Autodesk Fusion 360 part; units mm, degrees
(part 2 of 11)
  line L821 (19.8574, -105.4367) -> (19.8738, -105.4005)
  line L822 (-0.0787, -205.2079) -> (-0.0748, -205.2474)
  arc A58 (18.12, -106.7368) -> (18.4614, -106.8782) centre (18.32, -106.7368) ccw
  line L823 (0.0706, -205.5685) -> (0.0978, -205.5975)
  line L824 (19.7422, -105.5975) -> (19.7694, -105.5685)
  line L825 (0.0454, -45.5378) -> (0.0706, -45.5685)
  line L826 (19.9083, -105.2866) -> (19.9148, -105.2474)
  line L827 (-0.0338, -205.4005) -> (-0.0174, -205.4367)
  line L828 (19.7694, -105.5685) -> (19.7946, -105.5378)
  line L829 (1.72, -46.7368) -> (1.72, -44.4997)
  line L830 (19.9187, -105.2079) -> (19.92, -105.0997)
  line L831 (-0.0683, -45.2866) -> (-0.0593, -45.3253)
  arc A59 (1.3786, -46.8782) -> (1.72, -46.7368) centre (1.52, -46.7368) ccw
  line L832 (0.0706, -45.5685) -> (0.0978, -45.5975)
  line L833 (19.8387, -105.4717) -> (19.8574, -105.4367)
  line L834 (0.0454, -205.5378) -> (0.0706, -205.5685)
  line L835 (19.9148, -105.2474) -> (19.9187, -105.2079)
  line L836 (-0.0683, -205.2866) -> (-0.0593, -205.3253)
  line L837 (0.0223, -45.5055) -> (0.0454, -45.5378)
  line L838 (-0.0683, -45.2866) -> (-0.0593, -45.3253)
  line L839 (-0.0593, -45.3253) -> (-0.0478, -45.3633)
  line L840 (-0.0478, -185.3633) -> (-0.0338, -185.4005)
  line L841 (6.02, -189.7998) -> (6.2199, -189.9997)
  line L842 (9.713, -186.0997) -> (7.0807, -186.0997)
  line L843 (-0.0787, -205.2079) -> (-0.0748, -205.2474)
  line L844 (-0.0174, -45.4367) -> (0.0013, -45.4717)
  line L845 (19.9187, -105.2079) -> (19.92, -105.0997)
  line L846 (0.0706, -205.5685) -> (0.0978, -205.5975)
  line L847 (-0.0593, -45.3253) -> (-0.0478, -45.3633)
  line L848 (0.0454, -205.5378) -> (0.0706, -205.5685)
  line L849 (19.8993, -105.3253) -> (19.9083, -105.2866)
  line L850 (0.0223, -205.5055) -> (0.0454, -205.5378)
  line L851 (-0.0338, -205.4005) -> (-0.0174, -205.4367)
  line L852 (19.8177, -105.5055) -> (19.8387, -105.4717)
  line L853 (6.02, -187.1603) -> (6.02, -189.7998)
  line L854 (0.0013, -45.4717) -> (0.0223, -45.5055)
  line L855 (0.0223, -185.5055) -> (0.0454, -185.5378)
  line L856 (9.92, -186.3066) -> (9.713, -186.0997)
  line L857 (-0.0478, -45.3633) -> (-0.0338, -45.4005)
  line L858 (-0.08, -45.0997) -> (-0.0787, -45.2079)
  line L859 (19.8387, -105.4717) -> (19.8574, -105.4367)
  line L860 (0.0013, -205.4717) -> (0.0223, -205.5055)
  line L861 (19.7946, -105.5378) -> (19.8177, -105.5055)
  line L862 (19.9148, -105.2474) -> (19.9187, -105.2079)
  line L863 (19.8738, -105.4005) -> (19.8878, -105.3633)
  line L864 (1.72, -206.7368) -> (1.72, -204.4997)
  line L865 (-0.0593, -205.3253) -> (-0.0478, -205.3633)
  line L866 (19.8878, -105.3633) -> (19.8993, -105.3253)
  line L867 (19.8177, -105.5055) -> (19.8387, -105.4717)
  line L868 (-0.08, -185.0997) -> (-0.0787, -185.2079)
  line L869 (0.0013, -45.4717) -> (0.0223, -45.5055)
  line L870 (19.9083, -105.2866) -> (19.9148, -105.2474)
  line L871 (-0.0683, -205.2866) -> (-0.0593, -205.3253)
  line L872 (-0.0748, -205.2474) -> (-0.0683, -205.2866)
  line L873 (-0.0787, -45.2079) -> (-0.0748, -45.2474)
  line L874 (-0.0174, -205.4367) -> (0.0013, -205.4717)
  line L875 (18.4614, -106.8782) -> (19.7422, -105.5975)
  line L876 (-0.0174, -45.4367) -> (0.0013, -45.4717)
  line L877 (-0.0748, -205.2474) -> (-0.0683, -205.2866)
  line L878 (18.12, -97.2997) -> (18.12, -102.6997)
  line L879 (-0.08, -205.0997) -> (-0.0787, -205.2079)
  arc A60 (1.3786, -46.8782) -> (1.72, -46.7368) centre (1.52, -46.7368) ccw
  line L880 (10.127, -206.0997) -> (9.92, -206.3066)
  line L881 (-0.0593, -94.674) -> (-0.0683, -94.7127)
  line L882 (9.713, -193.8997) -> (9.92, -193.6927)
  circle A61 centre (9.92, -49.9997) radius 2.1
  line L883 (19.8878, -105.3633) -> (19.8993, -105.3253)
  line L884 (0.0223, -94.4938) -> (0.0013, -94.5276)
  line L885 (9.713, -206.0997) -> (7.0807, -206.0997)
  line L886 (10.127, -193.8997) -> (12.7593, -193.8997)
  line L887 (3.6807, -197.2997) -> (7.0807, -193.8997)
  line L888 (9.92, -193.6927) -> (10.127, -193.8997)
  line L889 (9.92, -206.3066) -> (9.713, -206.0997)
  line L890 (18.12, -102.6997) -> (16.1593, -102.6997)
  line L891 (16.4807, -104.4997) -> (18.12, -104.4997)
  line L892 (-0.0338, -45.4005) -> (-0.0174, -45.4367)
  line L893 (13.82, -107.1603) -> (16.4807, -104.4997)
  line L894 (7.0807, -206.0997) -> (3.6807, -202.6997)
  line L895 (7.0807, -193.8997) -> (9.713, -193.8997)
  line L896 (9.92, -206.3066) -> (9.713, -206.0997)
  line L897 (7.0807, -193.8997) -> (9.713, -193.8997)
  line L898 (19.8993, -105.3253) -> (19.9083, -105.2866)
  line L899 (-0.0174, -205.4367) -> (0.0013, -205.4717)
  line L900 (-0.08, -45.0997) -> (-0.0787, -45.2079)
  line L901 (0.0978, -45.5975) -> (1.3786, -46.8782)
  line L902 (6.02, -192.839) -> (3.3593, -195.4997)
  line L903 (10.127, -193.8997) -> (12.7593, -193.8997)
  line L904 (12.7593, -106.0997) -> (10.127, -106.0997)
  line L905 (-0.0338, -45.4005) -> (-0.0174, -45.4367)
  line L906 (0.0978, -45.5975) -> (1.3786, -46.8782)
  line L907 (-0.0748, -45.2474) -> (-0.0683, -45.2866)
  line L908 (13.82, -107.1603) -> (16.4807, -104.4997)
  line L909 (0.0013, -205.4717) -> (0.0223, -205.5055)
  line L910 (18.12, -97.2997) -> (18.12, -102.6997)
  line L911 (13.82, -109.7998) -> (13.82, -107.1603)
  line L912 (16.1593, -97.2997) -> (18.12, -97.2997)
  line L913 (-0.0478, -205.3633) -> (-0.0338, -205.4005)
  line L914 (0.0223, -45.5055) -> (0.0454, -45.5378)
  line L915 (18.12, -104.4997) -> (18.12, -106.7368)
  line L916 (16.1593, -102.6997) -> (12.7593, -106.0997)
  line L917 (-0.0478, -205.3633) -> (-0.0338, -205.4005)
  line L918 (-0.0478, -45.3633) -> (-0.0338, -45.4005)
  line L919 (18.12, -104.4997) -> (18.12, -106.7368)
  line L920 (6.02, -192.839) -> (3.3593, -195.4997)
  line L921 (19.7422, -105.5975) -> (19.7694, -105.5685)
  line L922 (12.7593, -106.0997) -> (10.127, -106.0997)
  line L923 (9.92, -193.6927) -> (10.127, -193.8997)
  line L924 (9.713, -193.8997) -> (9.92, -193.6927)
  line L925 (9.713, -206.0997) -> (7.0807, -206.0997)
  line L926 (12.7593, -206.0997) -> (10.127, -206.0997)
  line L927 (10.127, -206.0997) -> (9.92, -206.3066)
  line L928 (12.7593, -206.0997) -> (10.127, -206.0997)
  line L929 (13.82, -109.7998) -> (13.82, -107.1603)
  line L930 (-0.08, -194.8997) -> (-0.08, -205.0997)
  line L931 (-0.08, -194.8997) -> (-0.08, -205.0997)
  line L932 (18.12, -102.6997) -> (16.1593, -102.6997)
  line L933 (-0.0748, -45.2474) -> (-0.0683, -45.2866)
  line L934 (16.4807, -104.4997) -> (18.12, -104.4997)
  line L935 (16.1593, -97.2997) -> (18.12, -97.2997)
  line L936 (16.1593, -102.6997) -> (12.7593, -106.0997)
  line L937 (6.02, -47.1603) -> (6.02, -49.7998)
  line L938 (3.6807, -197.2997) -> (7.0807, -193.8997)
  line L939 (-0.0748, -94.7519) -> (-0.0787, -94.7914)
  line L940 (-0.0338, -94.5988) -> (-0.0478, -94.636)
  line L941 (3.3593, -95.4997) -> (1.72, -95.4997)
  line L942 (3.3593, -95.4997) -> (1.72, -95.4997)
  line L943 (-0.0593, -94.674) -> (-0.0683, -94.7127)
  line L944 (1.72, -204.4997) -> (3.3593, -204.4997)
  line L945 (1.72, -204.4997) -> (3.3593, -204.4997)
  line L946 (0.0706, -94.4308) -> (0.0454, -94.4616)
  line L947 (1.72, -197.2997) -> (3.6807, -197.2997)
  line L948 (3.6807, -202.6997) -> (1.72, -202.6997)
  line L949 (3.6807, -202.6997) -> (1.72, -202.6997)
  line L950 (0.0223, -94.4938) -> (0.0013, -94.5276)
  line L951 (0.0013, -94.5276) -> (-0.0174, -94.5626)
  line L952 (7.0807, -206.0997) -> (3.6807, -202.6997)
  line L953 (0.0223, -85.5055) -> (0.0454, -85.5378)
  line L954 (9.713, -53.8997) -> (9.92, -53.6927)
  line L955 (19.8738, -194.5988) -> (19.8574, -194.5626)
  arc A62 (1.3786, -86.8782) -> (1.72, -86.7368) centre (1.52, -86.7368) ccw
  line L956 (7.0807, -86.0997) -> (4.42, -83.439)
  line L957 (9.92, -53.6927) -> (10.127, -53.8997)
  line L958 (19.8574, -194.5626) -> (19.8387, -194.5276)
  line L959 (18.12, -204.4997) -> (18.12, -206.7368)
  line L960 (1.72, -84.4997) -> (3.3593, -84.4997)
  line L961 (0.0223, -85.5055) -> (0.0454, -85.5378)
  line L962 (7.0807, -86.0997) -> (4.42, -83.439)
  line L963 (19.8738, -194.5988) -> (19.8574, -194.5626)
  line L964 (-0.0748, -85.2474) -> (-0.0683, -85.2866)
  line L965 (-0.0338, -85.4005) -> (-0.0174, -85.4367)
  line L966 (19.7694, -194.4308) -> (19.7422, -194.4019)
  line L967 (19.9187, -194.7914) -> (19.9148, -194.7519)
  line L968 (0.0706, -85.5685) -> (0.0978, -85.5975)
  line L969 (-0.0338, -85.4005) -> (-0.0174, -85.4367)
  line L970 (3.3593, -84.4997) -> (6.02, -87.1603)
  line L971 (16.4807, -204.4997) -> (18.12, -204.4997)
  line L972 (9.92, -53.6927) -> (10.127, -53.8997)
  line L973 (19.9187, -205.2079) -> (19.92, -205.0997)
  line L974 (19.8738, -205.4005) -> (19.8878, -205.3633)
  line L975 (6.02, -52.839) -> (3.3593, -55.4997)
  line L976 (-0.0683, -85.2866) -> (-0.0593, -85.3253)
  line L977 (3.3593, -44.4997) -> (6.02, -47.1603)
  line L978 (-0.0478, -85.3633) -> (-0.0338, -85.4005)
  line L979 (19.9148, -194.7519) -> (19.9083, -194.7127)
  line L980 (18.12, -197.2997) -> (18.12, -202.6997)
  line L981 (0.0454, -85.5378) -> (0.0706, -85.5685)
  line L982 (18.12, -202.6997) -> (16.1593, -202.6997)
  line L983 (19.7946, -194.4616) -> (19.7694, -194.4308)
  line L984 (18.12, -202.6997) -> (16.1593, -202.6997)
  line L985 (6.02, -52.839) -> (3.3593, -55.4997)
  line L986 (6.02, -49.7998) -> (6.2199, -49.9997)
  line L987 (-0.0787, -85.2079) -> (-0.0748, -85.2474)
  arc A63 (1.3786, -86.8782) -> (1.72, -86.7368) centre (1.52, -86.7368) ccw
  line L988 (-0.0748, -85.2474) -> (-0.0683, -85.2866)
  line L989 (3.6807, -57.2997) -> (7.0807, -53.8997)
  line L990 (6.2199, -49.9997) -> (6.02, -50.1995)
  line L991 (-0.08, -85.0997) -> (-0.0787, -85.2079)
  line L992 (0.0706, -85.5685) -> (0.0978, -85.5975)
  line L993 (-0.0593, -85.3253) -> (-0.0478, -85.3633)
  line L994 (18.12, -197.2997) -> (18.12, -202.6997)
  line L995 (7.0807, -53.8997) -> (9.713, -53.8997)
  line L996 (10.127, -46.0997) -> (9.92, -46.3066)
  line L997 (0.0013, -85.4717) -> (0.0223, -85.5055)
  line L998 (16.1593, -197.2997) -> (18.12, -197.2997)
  line L999 (7.0807, -53.8997) -> (9.713, -53.8997)
  line L1000 (1.72, -84.4997) -> (3.3593, -84.4997)
  line L1001 (3.3593, -44.4997) -> (6.02, -47.1603)
  line L1002 (-0.0174, -85.4367) -> (0.0013, -85.4717)
  line L1003 (0.0454, -85.5378) -> (0.0706, -85.5685)
  line L1004 (18.12, -193.2625) -> (18.12, -195.4997)
  line L1005 (19.9083, -194.7127) -> (19.8993, -194.674)
  line L1006 (-0.0787, -85.2079) -> (-0.0748, -85.2474)
  line L1007 (-0.0174, -85.4367) -> (0.0013, -85.4717)
  line L1008 (16.1593, -197.2997) -> (18.12, -197.2997)
  line L1009 (0.0013, -85.4717) -> (0.0223, -85.5055)
  line L1010 (9.713, -46.0997) -> (7.0807, -46.0997)
  line L1011 (3.3593, -84.4997) -> (6.02, -87.1603)
  line L1012 (1.72, -86.7368) -> (1.72, -84.4997)
  line L1013 (6.02, -49.7998) -> (6.2199, -49.9997)
  line L1014 (1.72, -86.7368) -> (1.72, -84.4997)
  line L1015 (9.713, -93.8997) -> (9.92, -93.6927)
  line L1016 (19.8387, -205.4717) -> (19.8574, -205.4367)
  line L1017 (19.7946, -205.5378) -> (19.8177, -205.5055)
  line L1018 (19.9148, -205.2474) -> (19.9187, -205.2079)
  line L1019 (19.7422, -205.5975) -> (19.7694, -205.5685)
  line L1020 (13.6201, -89.9997) -> (13.82, -89.7998)
  line L1021 (10.127, -93.8997) -> (12.7593, -93.8997)
  line L1022 (18.12, -53.2625) -> (18.12, -55.4997)
  line L1023 (12.7593, -193.8997) -> (16.1593, -197.2997)
  line L1024 (18.12, -53.2625) -> (18.12, -55.4997)
  line L1025 (12.7593, -193.8997) -> (16.1593, -197.2997)
  line L1026 (1.72, -57.2997) -> (3.6807, -57.2997)
  line L1027 (10.127, -93.8997) -> (12.7593, -93.8997)
  line L1028 (19.92, -205.0997) -> (19.92, -194.8997)
  line L1029 (19.8878, -205.3633) -> (19.8993, -205.3253)
  line L1030 (19.7422, -205.5975) -> (19.7694, -205.5685)
  line L1031 (9.92, -46.3066) -> (9.713, -46.0997)
  line L1032 (19.8878, -205.3633) -> (19.8993, -205.3253)
  line L1033 (16.1593, -57.2997) -> (18.12, -57.2997)
  line L1034 (19.7422, -94.4019) -> (18.4614, -93.1211)
  line L1035 (19.8738, -205.4005) -> (19.8878, -205.3633)
  line L1036 (6.02, -87.1603) -> (6.02, -89.7998)
  line L1037 (19.7946, -205.5378) -> (19.8177, -205.5055)
  line L1038 (6.02, -50.1995) -> (6.02, -52.839)
  line L1039 (6.2199, -49.9997) -> (6.02, -50.1995)
  line L1040 (9.713, -53.8997) -> (9.92, -53.6927)
  line L1041 (6.02, -50.1995) -> (6.02, -52.839)
  line L1042 (3.6807, -57.2997) -> (7.0807, -53.8997)
  line L1043 (9.713, -46.0997) -> (7.0807, -46.0997)
  line L1044 (13.6201, -89.9997) -> (13.82, -89.7998)
  line L1045 (19.8993, -205.3253) -> (19.9083, -205.2866)
  line L1046 (19.8993, -205.3253) -> (19.9083, -205.2866)
  line L1047 (1.72, -44.4997) -> (3.3593, -44.4997)
  line L1048 (19.9083, -205.2866) -> (19.9148, -205.2474)
  line L1049 (19.7694, -205.5685) -> (19.7946, -205.5378)
  line L1050 (13.82, -90.1995) -> (13.6201, -89.9997)
  line L1051 (1.72, -44.4997) -> (3.3593, -44.4997)
  circle A64 centre (9.92, -49.9997) radius 2.1
  line L1052 (13.82, -90.1995) -> (13.6201, -89.9997)
  line L1053 (9.713, -93.8997) -> (9.92, -93.6927)
  line L1054 (3.3593, -55.4997) -> (1.72, -55.4997)
  line L1055 (19.8574, -205.4367) -> (19.8738, -205.4005)
  line L1056 (0.0978, -85.5975) -> (1.3786, -86.8782)
  line L1057 (19.8177, -205.5055) -> (19.8387, -205.4717)
  line L1058 (13.82, -92.839) -> (13.82, -90.1995)
  line L1059 (3.3593, -55.4997) -> (1.72, -55.4997)
  line L1060 (0.0978, -85.5975) -> (1.3786, -86.8782)
  line L1061 (9.92, -93.6927) -> (10.127, -93.8997)
  line L1062 (19.8387, -205.4717) -> (19.8574, -205.4367)
  line L1063 (19.8574, -205.4367) -> (19.8738, -205.4005)
  line L1064 (19.7694, -205.5685) -> (19.7946, -205.5378)
  line L1065 (19.9187, -205.2079) -> (19.92, -205.0997)
  line L1066 (13.82, -92.839) -> (13.82, -90.1995)
  line L1067 (18.12, -204.4997) -> (18.12, -206.7368)
  line L1068 (6.02, -87.1603) -> (6.02, -89.7998)
  line L1069 (19.8177, -205.5055) -> (19.8387, -205.4717)
  line L1070 (10.127, -46.0997) -> (9.92, -46.3066)
  line L1071 (19.9083, -205.2866) -> (19.9148, -205.2474)
  line L1072 (1.72, -57.2997) -> (3.6807, -57.2997)
  line L1073 (9.92, -93.6927) -> (10.127, -93.8997)
  line L1074 (19.9148, -205.2474) -> (19.9187, -205.2079)
  line L1075 (16.4807, -204.4997) -> (18.12, -204.4997)
  arc A65 (18.4614, -53.1211) -> (18.12, -53.2625) centre (18.32, -53.2625) ccw
  line L1076 (19.92, -205.0997) -> (19.92, -194.8997)
  line L1077 (16.4807, -55.4997) -> (13.82, -52.839)
  line L1078 (19.7946, -94.4616) -> (19.7694, -94.4308)
  line L1079 (16.4807, -95.4997) -> (13.82, -92.839)
  line L1080 (19.8738, -54.5988) -> (19.8574, -54.5626)
  line L1081 (6.02, -210.1995) -> (6.02, -212.839)
  line L1082 (19.7694, -54.4308) -> (19.7422, -54.4019)
  line L1083 (19.7422, -94.4019) -> (18.4614, -93.1211)
  line L1084 (0.0223, -214.4938) -> (0.0013, -214.5276)
  line L1085 (19.7946, -54.4616) -> (19.7694, -54.4308)
  arc A66 (1.72, -213.2625) -> (1.3786, -213.1211) centre (1.52, -213.2625) ccw
  line L1086 (18.12, -95.4997) -> (16.4807, -95.4997)
  line L1087 (19.92, -94.8997) -> (19.9187, -94.7914)
  line L1088 (19.9187, -94.7914) -> (19.9148, -94.7519)
  line L1089 (19.8993, -94.674) -> (19.8878, -94.636)
  line L1090 (16.1593, -57.2997) -> (18.12, -57.2997)
  line L1091 (18.12, -55.4997) -> (16.4807, -55.4997)
  line L1092 (19.8738, -94.5988) -> (19.8574, -94.5626)
  arc A67 (18.4614, -93.1211) -> (18.12, -93.2625) centre (18.32, -93.2625) ccw
  arc A68 (1.72, -213.2625) -> (1.3786, -213.1211) centre (1.52, -213.2625) ccw
  line L1093 (19.8574, -94.5626) -> (19.8387, -94.5276)
  line L1094 (19.9083, -94.7127) -> (19.8993, -94.674)
  line L1095 (19.92, -94.8997) -> (19.9187, -94.7914)
  line L1096 (19.7694, -94.4308) -> (19.7422, -94.4019)
  line L1097 (6.02, -207.1603) -> (6.02, -209.7998)
  line L1098 (18.12, -55.4997) -> (16.4807, -55.4997)
  line L1099 (19.8177, -94.4938) -> (19.7946, -94.4616)
  line L1100 (12.7593, -53.8997) -> (16.1593, -57.2997)
  line L1101 (19.8177, -54.4938) -> (19.7946, -54.4616)
  line L1102 (16.4807, -55.4997) -> (13.82, -52.839)
  line L1103 (19.9083, -94.7127) -> (19.8993, -94.674)
  line L1104 (16.1593, -202.6997) -> (12.7593, -206.0997)
  line L1105 (6.02, -207.1603) -> (6.02, -209.7998)
  line L1106 (16.1593, -202.6997) -> (12.7593, -206.0997)
  line L1107 (19.7694, -94.4308) -> (19.7422, -94.4019)
  line L1108 (18.12, -93.2625) -> (18.12, -95.4997)
  line L1109 (6.02, -209.7998) -> (6.2199, -209.9997)
  line L1110 (19.7946, -94.4616) -> (19.7694, -94.4308)
  line L1111 (19.8878, -94.636) -> (19.8738, -94.5988)
  line L1112 (19.8878, -94.636) -> (19.8738, -94.5988)
  line L1113 (19.8738, -94.5988) -> (19.8574, -94.5626)
  line L1114 (18.12, -93.2625) -> (18.12, -95.4997)
  line L1115 (19.7694, -54.4308) -> (19.7422, -54.4019)
  line L1116 (6.2199, -209.9997) -> (6.02, -210.1995)
  line L1117 (12.7593, -53.8997) -> (16.1593, -57.2997)
  line L1118 (19.8387, -94.5276) -> (19.8177, -94.4938)
  line L1119 (6.02, -209.7998) -> (6.2199, -209.9997)
  line L1120 (6.02, -210.1995) -> (6.02, -212.839)
  line L1121 (6.2199, -209.9997) -> (6.02, -210.1995)
  arc A69 (18.4614, -93.1211) -> (18.12, -93.2625) centre (18.32, -93.2625) ccw
  arc A70 (18.4614, -53.1211) -> (18.12, -53.2625) centre (18.32, -53.2625) ccw
  line L1122 (19.9148, -94.7519) -> (19.9083, -94.7127)
  line L1123 (19.92, -54.8997) -> (19.9187, -54.7914)
  line L1124 (18.12, -95.4997) -> (16.4807, -95.4997)
  line L1125 (19.8387, -94.5276) -> (19.8177, -94.4938)
  line L1126 (19.8993, -94.674) -> (19.8878, -94.636)
  line L1127 (19.8177, -94.4938) -> (19.7946, -94.4616)
  line L1128 (19.9148, -94.7519) -> (19.9083, -94.7127)
  line L1129 (19.9187, -94.7914) -> (19.9148, -94.7519)
  line L1130 (19.8574, -94.5626) -> (19.8387, -94.5276)
  line L1131 (16.4807, -95.4997) -> (13.82, -92.839)
  line L1132 (19.8387, -54.5276) -> (19.8177, -54.4938)
  line L1133 (0.0978, -214.4019) -> (0.0706, -214.4308)
  line L1134 (19.8993, -54.674) -> (19.8878, -54.636)
  line L1135 (19.7946, -54.4616) -> (19.7694, -54.4308)
  line L1136 (18.4614, -86.8782) -> (19.7422, -85.5975)
  line L1137 (19.92, -54.8997) -> (19.9187, -54.7914)
  line L1138 (19.8574, -54.5626) -> (19.8387, -54.5276)
  line L1139 (-0.0478, -214.636) -> (-0.0593, -214.674)
  line L1140 (0.0454, -214.4616) -> (0.0223, -214.4938)
  line L1141 (0.0013, -214.5276) -> (-0.0174, -214.5626)
  line L1142 (3.3593, -215.4997) -> (1.72, -215.4997)
  line L1143 (19.8177, -54.4938) -> (19.7946, -54.4616)
  line L1144 (19.7422, -85.5975) -> (19.7694, -85.5685)
  line L1145 (19.7694, -85.5685) -> (19.7946, -85.5378)
  line L1146 (3.3593, -215.4997) -> (1.72, -215.4997)
  line L1147 (16.4807, -84.4997) -> (18.12, -84.4997)
  line L1148 (18.12, -84.4997) -> (18.12, -86.7368)
  line L1149 (10.127, -86.0997) -> (9.92, -86.3066)
  line L1150 (12.7593, -86.0997) -> (10.127, -86.0997)
  line L1151 (19.9187, -85.2079) -> (19.92, -85.1682)
  line L1152 (19.8738, -85.4005) -> (19.8878, -85.3633)
  line L1153 (0.0706, -214.4308) -> (0.0454, -214.4616)
  arc A71 (18.12, -86.7368) -> (18.4614, -86.8782) centre (18.32, -86.7368) ccw
  line L1154 (15.42, -83.439) -> (12.7593, -86.0997)
  line L1155 (18.4614, -86.8782) -> (19.7422, -85.5975)
  line L1156 (-0.0338, -214.5988) -> (-0.0478, -214.636)
  line L1157 (19.7422, -85.5975) -> (19.7694, -85.5685)
  line L1158 (10.127, -86.0997) -> (9.92, -86.3066)
  arc A72 (18.12, -86.7368) -> (18.4614, -86.8782) centre (18.32, -86.7368) ccw
  line L1159 (12.7593, -86.0997) -> (10.127, -86.0997)
  line L1160 (0.0706, -214.4308) -> (0.0454, -214.4616)
  line L1161 (0.0978, -214.4019) -> (0.0706, -214.4308)
  line L1162 (-0.0174, -214.5626) -> (-0.0338, -214.5988)
  line L1163 (0.0454, -214.4616) -> (0.0223, -214.4938)
  line L1164 (-0.0593, -214.674) -> (-0.0683, -214.7127)
  line L1165 (15.42, -83.439) -> (12.7593, -86.0997)
  line L1166 (-0.0748, -214.7519) -> (-0.0787, -214.7914)
  line L1167 (-0.0478, -214.636) -> (-0.0593, -214.674)
  line L1168 (19.8993, -85.3253) -> (19.9083, -85.2866)
  line L1169 (-0.0174, -214.5626) -> (-0.0338, -214.5988)
  line L1170 (19.9148, -85.2474) -> (19.9187, -85.2079)
  line L1171 (9.92, -86.3066) -> (9.713, -86.0997)
  line L1172 (0.0223, -214.4938) -> (0.0013, -214.5276)
  line L1173 (19.8738, -85.4005) -> (19.8878, -85.3633)
  line L1174 (19.9187, -54.7914) -> (19.9148, -54.7519)
  line L1175 (9.92, -86.3066) -> (9.713, -86.0997)
  line L1176 (-0.0787, -214.7914) -> (-0.08, -214.8997)
  line L1177 (19.9187, -85.2079) -> (19.92, -85.1682)
  line L1178 (19.8878, -85.3633) -> (19.8993, -85.3253)
  line L1179 (19.8177, -85.5055) -> (19.8387, -85.4717)
  line L1180 (10.127, -186.0997) -> (9.92, -186.3066)
  line L1181 (19.7946, -85.5378) -> (19.8177, -85.5055)
  line L1182 (19.9148, -54.7519) -> (19.9083, -54.7127)
  line L1183 (-0.0593, -214.674) -> (-0.0683, -214.7127)
  line L1184 (-0.0683, -214.7127) -> (-0.0748, -214.7519)
  line L1185 (0.0013, -214.5276) -> (-0.0174, -214.5626)
  line L1186 (-0.0748, -214.7519) -> (-0.0787, -214.7914)
  line L1187 (19.7946, -85.5378) -> (19.8177, -85.5055)
  line L1188 (19.8993, -85.3253) -> (19.9083, -85.2866)
  line L1189 (-0.0683, -214.7127) -> (-0.0748, -214.7519)
  line L1190 (-0.0787, -214.7914) -> (-0.08, -214.8997)
  line L1191 (6.2199, -189.9997) -> (6.02, -190.1995)
  line L1192 (-0.0338, -214.5988) -> (-0.0478, -214.636)
  line L1193 (6.02, -170.1995) -> (6.02, -172.839)
  line L1194 (10.127, -186.0997) -> (9.92, -186.3066)
  line L1195 (18.12, -84.4997) -> (18.12, -86.7368)
  line L1196 (1.3786, -213.1211) -> (0.0978, -214.4019)
  line L1197 (6.2199, -169.9997) -> (6.02, -170.1995)
  arc A73 (-0.08, -219.4997) -> (0.42, -219.9997) centre (0.42, -219.4997) ccw
  line L1198 (1.42, -219.9997) -> (5.0886, -219.9997)
  line L1199 (19.8738, -54.5988) -> (19.8574, -54.5626)
  line L1200 (19.8574, -85.4367) -> (19.8738, -85.4005)
  line L1201 (6.02, -169.7998) -> (6.2199, -169.9997)
  line L1202 (9.713, -186.0997) -> (7.0807, -186.0997)
  line L1203 (6.02, -212.839) -> (3.3593, -215.4997)
  line L1204 (19.8878, -85.3633) -> (19.8993, -85.3253)
  line L1205 (7.0807, -186.0997) -> (3.6807, -182.6997)
  line L1206 (19.8177, -85.5055) -> (19.8387, -85.4717)
  line L1207 (19.9083, -85.2866) -> (19.9148, -85.2474)
  line L1208 (3.3593, -175.4997) -> (1.72, -175.4997)
  line L1209 (6.02, -170.1995) -> (6.02, -172.839)
  line L1210 (6.2199, -169.9997) -> (6.02, -170.1995)
  line L1211 (19.7694, -85.5685) -> (19.7946, -85.5378)
  line L1212 (19.8387, -54.5276) -> (19.8177, -54.4938)
  line L1213 (19.9187, -54.7914) -> (19.9148, -54.7519)
  line L1214 (19.8574, -85.4367) -> (19.8738, -85.4005)
  line L1215 (1.72, -215.4997) -> (1.72, -213.2625)
  line L1216 (19.8387, -85.4717) -> (19.8574, -85.4367)
  line L1217 (3.3593, -175.4997) -> (1.72, -175.4997)
  line L1218 (19.8387, -85.4717) -> (19.8574, -85.4367)
  line L1219 (6.02, -167.1603) -> (6.02, -169.7998)
  line L1220 (1.72, -186.7368) -> (1.72, -184.4997)
  line L1221 (19.9148, -85.2474) -> (19.9187, -85.2079)
  line L1222 (19.8993, -54.674) -> (19.8878, -54.636)
  line L1223 (19.8878, -54.636) -> (19.8738, -54.5988)
  line L1224 (19.8574, -54.5626) -> (19.8387, -54.5276)
  line L1225 (16.4807, -84.4997) -> (18.12, -84.4997)
  line L1226 (3.3593, -184.4997) -> (6.02, -187.1603)
  line L1227 (19.9083, -54.7127) -> (19.8993, -54.674)
  line L1228 (6.02, -212.839) -> (3.3593, -215.4997)
  line L1229 (1.72, -186.7368) -> (1.72, -184.4997)
  line L1230 (13.82, -87.1603) -> (16.4807, -84.4997)
  circle A74 centre (9.92, -89.9997) radius 2.1
  line L1231 (0.42, -219.9997) -> (1.42, -219.9997)
  line L1232 (19.9148, -54.7519) -> (19.9083, -54.7127)
  line L1233 (19.7422, -54.4019) -> (18.4614, -53.1211)
  line L1234 (3.3593, -184.4997) -> (6.02, -187.1603)
  line L1235 (0.42, -219.9997) -> (1.42, -219.9997)
  line L1236 (13.82, -89.7998) -> (13.82, -87.1603)
  line L1237 (6.02, -187.1603) -> (6.02, -189.7998)
  line L1238 (7.0807, -186.0997) -> (3.6807, -182.6997)
  line L1239 (19.7422, -54.4019) -> (18.4614, -53.1211)
  line L1240 (6.2199, -189.9997) -> (6.02, -190.1995)
  line L1241 (1.3786, -213.1211) -> (0.0978, -214.4019)
  line L1242 (1.72, -215.4997) -> (1.72, -213.2625)
  line L1243 (6.02, -189.7998) -> (6.2199, -189.9997)
  line L1244 (6.02, -172.839) -> (3.3593, -175.4997)
  line L1245 (6.02, -169.7998) -> (6.2199, -169.9997)
  line L1246 (13.82, -87.1603) -> (16.4807, -84.4997)
  line L1247 (19.9083, -54.7127) -> (19.8993, -54.674)
  line L1248 (19.9083, -85.2866) -> (19.9148, -85.2474)
  line L1249 (6.02, -172.839) -> (3.3593, -175.4997)
  line L1250 (9.92, -186.3066) -> (9.713, -186.0997)
  line L1251 (6.02, -167.1603) -> (6.02, -169.7998)
  circle A75 centre (9.92, -89.9997) radius 2.1
  line L1252 (19.8878, -54.636) -> (19.8738, -54.5988)
  line L1253 (13.82, -89.7998) -> (13.82, -87.1603)
  line L1254 (9.713, -86.0997) -> (7.0807, -86.0997)
  line L1255 (-0.08, -218.4997) -> (-0.08, -219.4997)
  line L1256 (7.0807, -93.8997) -> (9.713, -93.8997)
  line L1257 (4.42, -218.1997) -> (4.42, -216.5603)
  line L1258 (7.0807, -93.8997) -> (9.713, -93.8997)
  line L1259 (12.7593, -93.8997) -> (16.1593, -97.2997)
  line L1260 (9.92, -166.3066) -> (9.713, -166.0997)
  line L1261 (9.713, -86.0997) -> (7.0807, -86.0997)
  line L1262 (10.127, -166.0997) -> (9.92, -166.3066)
  line L1263 (9.92, -173.6927) -> (10.127, -173.8997)
  line L1264 (13.82, -172.839) -> (13.82, -170.1995)
  line L1265 (13.6201, -49.9997) -> (13.82, -49.7998)
  line L1266 (5.2457, -219.979) -> (5.2837, -219.9674)
  line L1267 (12.7593, -166.0997) -> (10.127, -166.0997)
  line L1268 (19.7946, -45.5378) -> (19.8177, -45.5055)
  line L1269 (19.7946, -45.5378) -> (19.8177, -45.5055)
  line L1270 (5.4888, -219.849) -> (5.5178, -219.8219)
  line L1271 (13.82, -172.839) -> (13.82, -170.1995)
  line L1272 (3.6807, -97.2997) -> (7.0807, -93.8997)
  line L1273 (-0.08, -218.4997) -> (-0.08, -219.4997)
  line L1274 (18.12, -182.6997) -> (16.1593, -182.6997)
  line L1275 (19.92, -105.0997) -> (19.92, -94.8997)
  line L1276 (-0.08, -94.8997) -> (-0.08, -105.0997)
  line L1277 (16.4807, -184.4997) -> (18.12, -184.4997)
  line L1278 (13.82, -49.7998) -> (13.82, -47.1603)
  line L1279 (10.127, -173.8997) -> (12.7593, -173.8997)
  line L1280 (5.3209, -219.9534) -> (5.357, -219.9371)
  line L1281 (18.12, -177.2997) -> (18.12, -182.6997)
  line L1282 (13.82, -170.1995) -> (13.6201, -169.9997)
  line L1283 (13.82, -50.1995) -> (13.6201, -49.9997)
  circle A76 centre (9.92, -169.9997) radius 2.1
  line L1284 (16.1593, -177.2997) -> (18.12, -177.2997)
  line L1285 (13.6201, -169.9997) -> (13.82, -169.7998)
  line L1286 (16.1593, -177.2997) -> (18.12, -177.2997)
  line L1287 (18.12, -182.6997) -> (16.1593, -182.6997)
  line L1288 (12.7593, -93.8997) -> (16.1593, -97.2997)
  line L1289 (13.82, -50.1995) -> (13.6201, -49.9997)
  arc A77 (-0.08, -219.4997) -> (0.42, -219.9997) centre (0.42, -219.4997) ccw
  line L1290 (9.92, -173.6927) -> (10.127, -173.8997)
  line L1291 (13.82, -169.7998) -> (13.82, -167.1603)
  line L1292 (9.92, -166.3066) -> (9.713, -166.0997)
  line L1293 (18.12, -177.2997) -> (18.12, -182.6997)
  line L1294 (13.82, -169.7998) -> (13.82, -167.1603)
  line L1295 (16.4807, -184.4997) -> (18.12, -184.4997)
  line L1296 (19.92, -105.0997) -> (19.92, -94.8997)
  line L1297 (5.3921, -219.9183) -> (5.4258, -219.8974)
  line L1298 (5.4258, -219.8974) -> (5.4581, -219.8742)
  line L1299 (5.1678, -219.9945) -> (5.207, -219.988)
  line L1300 (5.3921, -219.9183) -> (5.4258, -219.8974)
  line L1301 (18.4614, -186.8782) -> (19.7422, -185.5975)
  line L1302 (18.12, -44.4997) -> (18.12, -46.7368)
  line L1303 (1.42, -219.9997) -> (5.0886, -219.9997)
  line L1304 (13.82, -170.1995) -> (13.6201, -169.9997)
  line L1305 (5.2457, -219.979) -> (5.2837, -219.9674)
  line L1306 (19.8387, -45.4717) -> (19.8574, -45.4367)
  line L1307 (1.42, -79.9997) -> (0.42, -79.9997)
  line L1308 (4.42, -218.1997) -> (4.42, -216.5603)
  line L1309 (5.4258, -219.8974) -> (5.4581, -219.8742)
  line L1310 (10.127, -173.8997) -> (12.7593, -173.8997)
  line L1311 (13.82, -47.1603) -> (16.4807, -44.4997)
  line L1312 (13.6201, -49.9997) -> (13.82, -49.7998)
  line L1313 (13.82, -49.7998) -> (13.82, -47.1603)
  line L1314 (-0.08, -94.8997) -> (-0.08, -105.0997)
  line L1315 (13.82, -47.1603) -> (16.4807, -44.4997)
  line L1316 (3.6807, -97.2997) -> (7.0807, -93.8997)
  line L1317 (5.1283, -219.9984) -> (5.1678, -219.9945)
  line L1318 (12.7593, -166.0997) -> (10.127, -166.0997)
  line L1319 (19.9148, -185.2474) -> (19.9187, -185.2079)
  line L1320 (0.42, -79.9997) -> (1.42, -79.9997)
  line L1321 (1.42, -79.9997) -> (0.42, -79.9997)
  line L1322 (-0.08, -80.4997) -> (-0.08, -81.4997)
  arc A78 (18.12, -46.7368) -> (18.4614, -46.8782) centre (18.32, -46.7368) ccw
  line L1323 (5.357, -219.9371) -> (5.3921, -219.9183)
  line L1324 (18.4614, -46.8782) -> (19.7422, -45.5975)
  line L1325 (19.8738, -185.4005) -> (19.8878, -185.3633)
  line L1326 (19.7422, -185.5975) -> (19.7694, -185.5685)
  line L1327 (19.8738, -45.4005) -> (19.8878, -45.3633)
  line L1328 (5.4581, -219.8742) -> (5.4888, -219.849)
  line L1329 (19.8574, -45.4367) -> (19.8738, -45.4005)
  line L1330 (1.42, -79.9997) -> (5.0886, -79.9997)
  line L1331 (19.7694, -185.5685) -> (19.7946, -185.5378)
  line L1332 (5.3209, -219.9534) -> (5.357, -219.9371)
  line L1333 (19.8993, -185.3253) -> (19.9083, -185.2866)
  line L1334 (5.207, -219.988) -> (5.2457, -219.979)
  arc A79 (6.6572, -81.7997) -> (6.7986, -81.4582) centre (6.6572, -81.5997) ccw
  line L1335 (0.42, -79.9997) -> (1.42, -79.9997)
  line L1336 (19.8878, -185.3633) -> (19.8993, -185.3253)
  line L1337 (5.5178, -219.8219) -> (6.7986, -218.5411)
  arc A80 (-0.08, -79.4997) -> (0.42, -79.9997) centre (0.42, -79.4997) ccw
  line L1338 (19.8878, -45.3633) -> (19.8993, -45.3253)
  arc A81 (18.12, -46.7368) -> (18.4614, -46.8782) centre (18.32, -46.7368) ccw
  arc A82 (6.6572, -81.7997) -> (6.7986, -81.4582) centre (6.6572, -81.5997) ccw
  line L1339 (19.9148, -185.2474) -> (19.9187, -185.2079)
  line L1340 (6.7986, -81.4582) -> (5.5178, -80.1775)
  line L1341 (19.9187, -45.2079) -> (19.92, -45.0997)
  line L1342 (19.8878, -185.3633) -> (19.8993, -185.3253)
  line L1343 (5.4888, -219.849) -> (5.5178, -219.8219)
  line L1344 (19.9083, -45.2866) -> (19.9148, -45.2474)
  line L1345 (19.9187, -185.2079) -> (19.92, -185.0997)
  line L1346 (-0.08, -80.4997) -> (-0.08, -81.4997)
  line L1347 (19.8738, -45.4005) -> (19.8878, -45.3633)
  line L1348 (19.7422, -45.5975) -> (19.7694, -45.5685)
  line L1349 (13.6201, -169.9997) -> (13.82, -169.7998)
  arc A83 (6.7986, -218.5411) -> (6.6572, -218.1997) centre (6.6572, -218.3997) ccw
  line L1350 (5.1678, -219.9945) -> (5.207, -219.988)
  arc A84 (0.42, -79.9997) -> (-0.08, -80.4997) centre (0.42, -80.4997) ccw
  line L1351 (19.7422, -185.5975) -> (19.7694, -185.5685)
  line L1352 (1.42, -79.9997) -> (5.0886, -79.9997)
  line L1353 (19.8387, -185.4717) -> (19.8574, -185.4367)
  line L1354 (5.0886, -79.9997) -> (1.42, -79.9997)
  arc A85 (-0.08, -79.4997) -> (0.42, -79.9997) centre (0.42, -79.4997) ccw
  line L1355 (19.8177, -45.5055) -> (19.8387, -45.4717)
  line L1356 (9.713, -173.8997) -> (9.92, -173.6927)
  line L1357 (19.8387, -45.4717) -> (19.8574, -45.4367)
  line L1358 (9.713, -173.8997) -> (9.92, -173.6927)
  line L1359 (19.7946, -185.5378) -> (19.8177, -185.5055)
  line L1360 (19.9083, -45.2866) -> (19.9148, -45.2474)
  line L1361 (5.2837, -219.9674) -> (5.3209, -219.9534)
  arc A86 (0.42, -79.9997) -> (-0.08, -80.4997) centre (0.42, -80.4997) ccw
  line L1362 (19.7946, -185.5378) -> (19.8177, -185.5055)
  line L1363 (5.207, -219.988) -> (5.2457, -219.979)
  line L1364 (19.9083, -185.2866) -> (19.9148, -185.2474)
  line L1365 (19.9083, -185.2866) -> (19.9148, -185.2474)
  line L1366 (19.7694, -185.5685) -> (19.7946, -185.5378)
  circle A87 centre (9.92, -169.9997) radius 2.1
  arc A88 (6.7986, -218.5411) -> (6.6572, -218.1997) centre (6.6572, -218.3997) ccw
  line L1367 (10.127, -166.0997) -> (9.92, -166.3066)
  line L1368 (19.8993, -45.3253) -> (19.9083, -45.2866)
  line L1369 (5.0886, -79.9997) -> (1.42, -79.9997)
  line L1370 (5.2837, -219.9674) -> (5.3209, -219.9534)
  line L1371 (18.12, -44.4997) -> (18.12, -46.7368)
  line L1372 (5.357, -219.9371) -> (5.3921, -219.9183)
  line L1373 (5.4581, -219.8742) -> (5.4888, -219.849)
  line L1374 (6.7986, -81.4582) -> (5.5178, -80.1775)
  line L1375 (19.8878, -165.3633) -> (19.8993, -165.3253)
  line L1376 (19.9148, -45.2474) -> (19.9187, -45.2079)
  line L1377 (19.7946, -165.5378) -> (19.8177, -165.5055)
  line L1378 (19.7694, -45.5685) -> (19.7946, -45.5378)
  line L1379 (5.5178, -219.8219) -> (6.7986, -218.5411)
  line L1380 (18.4614, -186.8782) -> (19.7422, -185.5975)
  line L1381 (5.1283, -219.9984) -> (5.1678, -219.9945)
  line L1382 (19.7694, -45.5685) -> (19.7946, -45.5378)
  line L1383 (19.8993, -185.3253) -> (19.9083, -185.2866)
  line L1384 (6.6572, -218.1997) -> (4.42, -218.1997)
  line L1385 (19.8738, -165.4005) -> (19.8878, -165.3633)
  line L1386 (19.8574, -185.4367) -> (19.8738, -185.4005)
  line L1387 (14.4479, -80.081) -> (14.4142, -80.102)
  line L1388 (14.483, -79.9371) -> (14.5191, -79.9534)
  line L1389 (14.3819, -79.8742) -> (14.4142, -79.8974)
  line L1390 (14.483, -80.0623) -> (14.4479, -80.081)
  line L1391 (19.8878, -34.636) -> (19.8738, -34.5988)
  line L1392 (19.7422, -34.4019) -> (18.4614, -33.1211)
  line L1393 (19.9148, -34.7519) -> (19.9083, -34.7127)
  line L1394 (12.7593, -33.8997) -> (16.1593, -37.2997)
  line L1395 (12.7593, -33.8997) -> (16.1593, -37.2997)
  line L1396 (13.82, -207.1603) -> (16.4807, -204.4997)
  line L1397 (16.4807, -35.4997) -> (13.82, -32.839)
  line L1398 (14.483, -79.9371) -> (14.5191, -79.9534)
  line L1399 (7.0807, -33.8997) -> (9.713, -33.8997)
  line L1400 (13.82, -207.1603) -> (16.4807, -204.4997)
  line L1401 (19.8177, -34.4938) -> (19.7946, -34.4616)
  line L1402 (19.9187, -34.7914) -> (19.9148, -34.7519)
  line L1403 (14.3819, -80.1251) -> (14.3512, -80.1503)
  line L1404 (7.0807, -213.8997) -> (9.7152, -213.8997)
  line L1405 (19.8387, -34.5276) -> (19.8177, -34.4938)
  line L1406 (16.1593, -37.2997) -> (18.12, -37.2997)
  line L1407 (19.8387, -34.5276) -> (19.8177, -34.4938)
  line L1408 (19.9187, -34.7914) -> (19.9148, -34.7519)
  line L1409 (19.8574, -34.5626) -> (19.8387, -34.5276)
  line L1410 (12.7593, -213.8997) -> (15.42, -216.5603)
  arc A89 (18.4614, -33.1211) -> (18.12, -33.2625) centre (18.32, -33.2625) ccw
  line L1411 (14.3512, -80.1503) -> (14.3222, -80.1775)
  line L1412 (14.5191, -80.0459) -> (14.483, -80.0623)
  line L1413 (18.4614, -206.8782) -> (19.7422, -205.5975)
  line L1414 (19.7422, -214.4019) -> (18.4614, -213.1211)
  line L1415 (18.12, -213.2625) -> (18.12, -215.4997)
  line L1416 (14.3819, -80.1251) -> (14.3512, -80.1503)
  line L1417 (14.4479, -79.9183) -> (14.483, -79.9371)
  line L1418 (19.7946, -34.4616) -> (19.7694, -34.4308)
  line L1419 (14.3222, -79.8219) -> (14.3512, -79.849)
  line L1420 (18.12, -33.2625) -> (18.12, -35.4997)
  line L1421 (14.4142, -79.8974) -> (14.4479, -79.9183)
  line L1422 (19.8878, -34.636) -> (19.8738, -34.5988)
  line L1423 (14.4479, -80.081) -> (14.4142, -80.102)
  line L1424 (14.483, -80.0623) -> (14.4479, -80.081)
  line L1425 (16.4807, -215.4997) -> (13.82, -212.839)
  line L1426 (14.3512, -79.849) -> (14.3819, -79.8742)
  line L1427 (18.12, -35.4997) -> (16.4807, -35.4997)
  line L1428 (14.4479, -79.9183) -> (14.483, -79.9371)
  line L1429 (14.4142, -79.8974) -> (14.4479, -79.9183)
  line L1430 (19.8993, -34.674) -> (19.8878, -34.636)
  arc A90 (1.3786, -206.8782) -> (1.72, -206.7368) centre (1.52, -206.7368) ccw
  line L1431 (14.3512, -79.849) -> (14.3819, -79.8742)
  line L1432 (18.12, -37.2997) -> (18.12, -42.6997)
  line L1433 (19.9148, -34.7519) -> (19.9083, -34.7127)
  line L1434 (14.3512, -80.1503) -> (14.3222, -80.1775)
  line L1435 (14.4142, -80.102) -> (14.3819, -80.1251)
  line L1436 (14.3222, -79.8219) -> (14.3512, -79.849)
  line L1437 (14.5191, -80.0459) -> (14.483, -80.0623)
  line L1438 (19.7422, -34.4019) -> (18.4614, -33.1211)
  line L1439 (7.0807, -213.8997) -> (9.7152, -213.8997)
  arc A91 (18.12, -206.7368) -> (18.4614, -206.8782) centre (18.32, -206.7368) ccw
  line L1440 (0.0978, -205.5975) -> (1.3786, -206.8782)
  line L1441 (19.8993, -34.674) -> (19.8878, -34.636)
  line L1442 (14.3819, -79.8742) -> (14.4142, -79.8974)
  line L1443 (14.4142, -80.102) -> (14.3819, -80.1251)
  line L1444 (19.7946, -34.4616) -> (19.7694, -34.4308)
  line L1445 (19.7694, -34.4308) -> (19.7422, -34.4019)
  line L1446 (19.92, -34.8997) -> (19.9187, -34.7914)
  line L1447 (16.4807, -35.4997) -> (13.82, -32.839)
  line L1448 (18.12, -162.6997) -> (16.1593, -162.6997)
  line L1449 (19.8177, -185.5055) -> (19.8387, -185.4717)
  line L1450 (19.8574, -185.4367) -> (19.8738, -185.4005)
  arc A92 (18.12, -166.7368) -> (18.4614, -166.8782) centre (18.32, -166.7368) ccw
  line L1451 (5.207, -80.0113) -> (5.1678, -80.0049)
  line L1452 (19.8738, -185.4005) -> (19.8878, -185.3633)
  line L1453 (13.82, -190.1995) -> (13.6201, -189.9997)
  line L1454 (5.207, -80.0113) -> (5.1678, -80.0049)
  line L1455 (18.4614, -166.8782) -> (19.7422, -165.5975)
  line L1456 (13.82, -190.1995) -> (13.6201, -189.9997)
  line L1457 (5.0886, -219.9997) -> (5.1283, -219.9984)
  line L1458 (5.207, -79.988) -> (5.2457, -79.979)
  line L1459 (5.2837, -80.0319) -> (5.2457, -80.0203)
  line L1460 (19.9148, -45.2474) -> (19.9187, -45.2079)
  line L1461 (19.8574, -165.4367) -> (19.8738, -165.4005)
  line L1462 (10.127, -53.8997) -> (12.7593, -53.8997)
  line L1463 (5.1678, -80.0049) -> (5.1283, -80.001)
  line L1464 (13.82, -189.7998) -> (13.82, -187.1603)
  line L1465 (13.6201, -189.9997) -> (13.82, -189.7998)
  line L1466 (16.4807, -164.4997) -> (18.12, -164.4997)
  line L1467 (5.2457, -79.979) -> (5.2837, -79.9674)
  line L1468 (13.6201, -189.9997) -> (13.82, -189.7998)
  line L1469 (19.8738, -165.4005) -> (19.8878, -165.3633)
  line L1470 (19.8574, -45.4367) -> (19.8738, -45.4005)
  line L1471 (13.82, -52.839) -> (13.82, -50.1995)
  line L1472 (12.7593, -46.0997) -> (10.127, -46.0997)
  line L1473 (19.7694, -165.5685) -> (19.7946, -165.5378)
  line L1474 (19.8574, -165.4367) -> (19.8738, -165.4005)
  line L1475 (13.82, -189.7998) -> (13.82, -187.1603)
  line L1476 (10.127, -53.8997) -> (12.7593, -53.8997)
  line L1477 (18.12, -162.6997) -> (16.1593, -162.6997)
  arc A93 (18.12, -186.7368) -> (18.4614, -186.8782) centre (18.32, -186.7368) ccw
  line L1478 (16.4807, -44.4997) -> (18.12, -44.4997)
  line L1479 (6.6572, -218.1997) -> (4.42, -218.1997)
  line L1480 (19.8878, -165.3633) -> (19.8993, -165.3253)
  line L1481 (19.8177, -185.5055) -> (19.8387, -185.4717)
  line L1482 (19.8387, -165.4717) -> (19.8574, -165.4367)
  line L1483 (-0.08, -214.8997) -> (-0.08, -218.4997)
  line L1484 (19.7422, -45.5975) -> (19.7694, -45.5685)
  line L1485 (19.8993, -45.3253) -> (19.9083, -45.2866)
  line L1486 (18.4614, -46.8782) -> (19.7422, -45.5975)
  line L1487 (19.7694, -165.5685) -> (19.7946, -165.5378)
  line L1488 (5.0886, -219.9997) -> (5.1283, -219.9984)
  line L1489 (5.2457, -80.0203) -> (5.207, -80.0113)
  line L1490 (5.1678, -79.9945) -> (5.207, -79.988)
  line L1491 (4.42, -216.5603) -> (7.0807, -213.8997)
  line L1492 (4.42, -216.5603) -> (7.0807, -213.8997)
  line L1493 (19.9187, -185.2079) -> (19.92, -185.0997)
  line L1494 (5.2457, -80.0203) -> (5.207, -80.0113)
  line L1495 (5.1283, -79.9984) -> (5.1678, -79.9945)
  line L1496 (19.8387, -185.4717) -> (19.8574, -185.4367)
  line L1497 (5.2457, -79.979) -> (5.2837, -79.9674)
  line L1498 (16.4807, -44.4997) -> (18.12, -44.4997)
  line L1499 (19.9187, -45.2079) -> (19.92, -45.0997)
  arc A94 (18.12, -186.7368) -> (18.4614, -186.8782) centre (18.32, -186.7368) ccw
  line L1500 (18.12, -164.4997) -> (18.12, -166.7368)
  line L1501 (19.8177, -45.5055) -> (19.8387, -45.4717)
  line L1502 (19.8878, -45.3633) -> (19.8993, -45.3253)
  line L1503 (-0.08, -214.8997) -> (-0.08, -218.4997)
  line L1504 (5.1678, -79.9945) -> (5.207, -79.988)
  line L1505 (19.7422, -165.5975) -> (19.7694, -165.5685)
  line L1506 (5.207, -79.988) -> (5.2457, -79.979)
  line L1507 (13.82, -52.839) -> (13.82, -50.1995)
  line L1508 (19.9083, -165.2866) -> (19.9148, -165.2474)
  line L1509 (19.7946, -165.5378) -> (19.8177, -165.5055)
  line L1510 (12.7593, -46.0997) -> (10.127, -46.0997)
  line L1511 (3.3593, -35.4997) -> (1.72, -35.4997)
  line L1512 (1.72, -42.6997) -> (1.72, -37.2997)
  line L1513 (19.9148, -165.2474) -> (19.9187, -165.2079)
  line L1514 (19.8177, -165.5055) -> (19.8387, -165.4717)
  line L1515 (9.7152, -213.8997) -> (9.92, -213.6949)
  circle A95 centre (9.92, -209.9997) radius 2.1
  line L1516 (16.1593, -182.6997) -> (12.7593, -186.0997)
  line L1517 (13.82, -187.1603) -> (16.4807, -184.4997)
  arc A96 (18.12, -166.7368) -> (18.4614, -166.8782) centre (18.32, -166.7368) ccw
  line L1518 (9.92, -213.6949) -> (10.127, -213.8997)
  line L1519 (19.8993, -165.3253) -> (19.9083, -165.2866)
  line L1520 (10.127, -213.8997) -> (12.7593, -213.8997)
  line L1521 (5.2837, -80.0319) -> (5.2457, -80.0203)
  line L1522 (19.9187, -165.2079) -> (19.92, -165.0997)
  line L1523 (19.7422, -165.5975) -> (19.7694, -165.5685)
  line L1524 (18.12, -184.4997) -> (18.12, -186.7368)
  arc A97 (18.4614, -213.1211) -> (18.12, -213.2625) centre (18.32, -213.2625) ccw
  arc A98 (18.4614, -213.1211) -> (18.12, -213.2625) centre (18.32, -213.2625) ccw
  line L1525 (1.72, -42.6997) -> (1.72, -37.2997)
  line L1526 (5.4258, -80.102) -> (5.3921, -80.081)
  line L1527 (5.4888, -80.1503) -> (5.4581, -80.1251)
  line L1528 (10.127, -213.8997) -> (12.7593, -213.8997)
  line L1529 (5.3209, -79.9534) -> (5.357, -79.9371)
  line L1530 (5.3209, -79.9534) -> (5.357, -79.9371)
  line L1531 (9.92, -213.6949) -> (10.127, -213.8997)
  line L1532 (5.3921, -80.081) -> (5.357, -80.0623)
  line L1533 (19.9187, -165.2079) -> (19.92, -165.0997)
  line L1534 (19.9148, -165.2474) -> (19.9187, -165.2079)
  line L1535 (5.1678, -80.0049) -> (5.1283, -80.001)
  line L1536 (18.12, -184.4997) -> (18.12, -186.7368)
  line L1537 (19.8993, -165.3253) -> (19.9083, -165.2866)
  line L1538 (12.7593, -186.0997) -> (10.127, -186.0997)
  line L1539 (5.357, -80.0623) -> (5.3209, -80.0459)
  line L1540 (9.7152, -213.8997) -> (9.92, -213.6949)
  line L1541 (3.3593, -35.4997) -> (1.72, -35.4997)
  line L1542 (5.357, -80.0623) -> (5.3209, -80.0459)
  line L1543 (16.1593, -182.6997) -> (12.7593, -186.0997)
  line L1544 (5.1283, -79.9984) -> (5.1678, -79.9945)
  line L1545 (13.6201, -209.9997) -> (13.82, -209.7998)
  line L1546 (5.4581, -80.1251) -> (5.4258, -80.102)
  line L1547 (13.82, -209.7998) -> (13.82, -207.1603)
  line L1548 (5.4258, -79.8974) -> (5.4581, -79.8742)
  line L1549 (13.82, -187.1603) -> (16.4807, -184.4997)
  line L1550 (13.82, -210.1995) -> (13.6201, -209.9997)
  line L1551 (5.4888, -80.1503) -> (5.4581, -80.1251)
  line L1552 (5.4581, -79.8742) -> (5.4888, -79.849)
  line L1553 (19.8387, -165.4717) -> (19.8574, -165.4367)
  line L1554 (16.4807, -164.4997) -> (18.12, -164.4997)
  line L1555 (18.12, -164.4997) -> (18.12, -166.7368)
  line L1556 (5.4258, -79.8974) -> (5.4581, -79.8742)
  line L1557 (13.82, -210.1995) -> (13.6201, -209.9997)
  line L1558 (1.72, -37.2997) -> (3.6807, -37.2997)
  line L1559 (1.72, -37.2997) -> (3.6807, -37.2997)
  line L1560 (12.7593, -186.0997) -> (10.127, -186.0997)
  line L1561 (3.6807, -42.6997) -> (1.72, -42.6997)
  line L1562 (19.8177, -165.5055) -> (19.8387, -165.4717)
  line L1563 (13.82, -209.7998) -> (13.82, -207.1603)
  line L1564 (18.4614, -166.8782) -> (19.7422, -165.5975)
  circle A99 centre (9.92, -209.9997) radius 2.1
  line L1565 (19.9083, -165.2866) -> (19.9148, -165.2474)
  line L1566 (3.6807, -42.6997) -> (1.72, -42.6997)
  line L1567 (13.82, -212.839) -> (13.82, -210.1995)
  line L1568 (5.3921, -80.081) -> (5.357, -80.0623)
  line L1569 (19.8574, -174.5626) -> (19.8387, -174.5276)
  line L1570 (4.42, -81.7997) -> (6.6572, -81.7997)
  line L1571 (13.82, -212.839) -> (13.82, -210.1995)
  line L1572 (0.0454, -34.4616) -> (0.0223, -34.4938)
  line L1573 (19.7422, -174.4019) -> (18.4614, -173.1211)
  line L1574 (0.0978, -34.4019) -> (0.0706, -34.4308)
  line L1575 (-0.0683, -34.7127) -> (-0.0748, -34.7519)
  line L1576 (5.0886, -79.9997) -> (5.1283, -79.9984)
  line L1577 (5.2837, -79.9674) -> (5.3209, -79.9534)
  line L1578 (19.7694, -174.4308) -> (19.7422, -174.4019)
  line L1579 (5.0886, -79.9997) -> (5.1283, -79.9984)
  line L1580 (5.3921, -79.9183) -> (5.4258, -79.8974)
  line L1581 (19.8387, -174.5276) -> (19.8177, -174.4938)
  line L1582 (-0.0174, -34.5626) -> (-0.0338, -34.5988)
  line L1583 (13.6201, -209.9997) -> (13.82, -209.7998)
  line L1584 (5.5178, -80.1775) -> (5.4888, -80.1503)
  line L1585 (-0.0478, -34.636) -> (-0.0593, -34.674)
  line L1586 (-0.0593, -34.674) -> (-0.0683, -34.7127)
  line L1587 (0.0223, -34.4938) -> (0.0013, -34.5276)
  line L1588 (-0.0787, -34.7914) -> (-0.08, -34.8997)
  line L1589 (5.4581, -80.1251) -> (5.4258, -80.102)
  line L1590 (14.5943, -219.979) -> (14.633, -219.988)
  line L1591 (14.4479, -219.9183) -> (14.483, -219.9371)
  line L1592 (19.9083, -174.7127) -> (19.8993, -174.674)
  line L1593 (5.2837, -79.9674) -> (5.3209, -79.9534)
  line L1594 (5.3209, -80.0459) -> (5.2837, -80.0319)
  line L1595 (5.357, -79.9371) -> (5.3921, -79.9183)
  line L1596 (5.4581, -79.8742) -> (5.4888, -79.849)
  arc A100 (1.72, -33.2625) -> (1.3786, -33.1211) centre (1.52, -33.2625) ccw
  line L1597 (19.8177, -174.4938) -> (19.7946, -174.4616)
  line L1598 (1.3786, -33.1211) -> (0.0978, -34.4019)
  line L1599 (5.4888, -79.849) -> (5.5178, -79.8219)
  line L1600 (19.7422, -174.4019) -> (18.4614, -173.1211)
  line L1601 (5.3209, -80.0459) -> (5.2837, -80.0319)
  line L1602 (5.5178, -80.1775) -> (5.4888, -80.1503)
  line L1603 (18.12, -175.4997) -> (16.4807, -175.4997)
  line L1604 (18.12, -173.2625) -> (18.12, -175.4997)
  line L1605 (5.4258, -80.102) -> (5.3921, -80.081)
  line L1606 (14.7117, -219.9984) -> (14.7514, -219.9997)
  line L1607 (14.4142, -219.8974) -> (14.4479, -219.9183)
  line L1608 (-0.0683, -34.7127) -> (-0.0748, -34.7519)
  line L1609 (14.4142, -219.8974) -> (14.4479, -219.9183)
  line L1610 (14.5191, -219.9534) -> (14.5563, -219.9674)
  line L1611 (5.1283, -80.001) -> (5.0886, -79.9997)
  line L1612 (-0.0787, -34.7914) -> (-0.08, -34.8997)
  line L1613 (-0.0748, -34.7519) -> (-0.0787, -34.7914)
  arc A101 (13.1828, -218.1997) -> (13.0414, -218.5411) centre (13.1828, -218.3997) ccw
  line L1614 (5.357, -79.9371) -> (5.3921, -79.9183)
  line L1615 (1.3786, -33.1211) -> (0.0978, -34.4019)
  line L1616 (5.3921, -79.9183) -> (5.4258, -79.8974)
  line L1617 (5.4888, -79.849) -> (5.5178, -79.8219)
  line L1618 (19.7694, -174.4308) -> (19.7422, -174.4019)
  line L1619 (5.1283, -80.001) -> (5.0886, -79.9997)
  line L1620 (0.0013, -34.5276) -> (-0.0174, -34.5626)
  line L1621 (0.0223, -34.4938) -> (0.0013, -34.5276)
  line L1622 (14.5563, -219.9674) -> (14.5943, -219.979)
  line L1623 (4.42, -81.7997) -> (6.6572, -81.7997)
  line L1624 (-0.0338, -34.5988) -> (-0.0478, -34.636)
  line L1625 (-0.0748, -34.7519) -> (-0.0787, -34.7914)
  line L1626 (19.7946, -174.4616) -> (19.7694, -174.4308)
  arc A102 (1.72, -33.2625) -> (1.3786, -33.1211) centre (1.52, -33.2625) ccw
  line L1627 (14.6722, -219.9945) -> (14.7117, -219.9984)
  line L1628 (13.0414, -218.5411) -> (14.3222, -219.8219)
  line L1629 (19.8177, -174.4938) -> (19.7946, -174.4616)
  line L1630 (14.633, -219.988) -> (14.6722, -219.9945)
  line L1631 (14.3222, -219.8219) -> (14.3512, -219.849)
  line L1632 (0.0706, -34.4308) -> (0.0454, -34.4616)
  line L1633 (19.8878, -174.636) -> (19.8738, -174.5988)
  line L1634 (6.02, -29.7998) -> (6.2199, -29.9997)
  line L1635 (-0.0748, -74.7519) -> (-0.0787, -74.7914)
  line L1636 (14.7117, -219.9984) -> (14.7514, -219.9997)
  line L1637 (-0.0174, -34.5626) -> (-0.0338, -34.5988)
  line L1638 (0.0978, -34.4019) -> (0.0706, -34.4308)
  line L1639 (14.5191, -219.9534) -> (14.5563, -219.9674)
  line L1640 (15.42, -216.5603) -> (15.42, -218.1997)
  line L1641 (6.02, -27.1603) -> (6.02, -29.7998)
  line L1642 (0.0706, -34.4308) -> (0.0454, -34.4616)
  line L1643 (19.92, -174.8997) -> (19.9187, -174.7914)
  line L1644 (-0.0593, -34.674) -> (-0.0683, -34.7127)
  line L1645 (6.2199, -29.9997) -> (6.02, -30.1995)
  line L1646 (14.6722, -219.9945) -> (14.7117, -219.9984)
  arc A103 (18.4614, -173.1211) -> (18.12, -173.2625) centre (18.32, -173.2625) ccw
  line L1647 (6.02, -30.1995) -> (6.02, -32.839)
  line L1648 (19.92, -174.8997) -> (19.9187, -174.7914)
  line L1649 (14.633, -219.988) -> (14.6722, -219.9945)
  line L1650 (0.0013, -34.5276) -> (-0.0174, -34.5626)
  line L1651 (19.8878, -174.636) -> (19.8738, -174.5988)
  line L1652 (0.0454, -34.4616) -> (0.0223, -34.4938)
  line L1653 (15.42, -218.1997) -> (13.1828, -218.1997)
  line L1654 (19.9187, -174.7914) -> (19.9148, -174.7519)
  line L1655 (-0.0478, -34.636) -> (-0.0593, -34.674)
  line L1656 (14.3819, -219.8742) -> (14.4142, -219.8974)
  line L1657 (14.5563, -219.9674) -> (14.5943, -219.979)
  line L1658 (19.9187, -174.7914) -> (19.9148, -174.7519)
  line L1659 (-0.0787, -74.7914) -> (-0.08, -74.8997)
  line L1660 (0.0223, -74.4938) -> (0.0013, -74.5276)
  line L1661 (19.8993, -174.674) -> (19.8878, -174.636)
  line L1662 (0.0013, -74.5276) -> (-0.0174, -74.5626)
  line L1663 (14.3222, -219.8219) -> (14.3512, -219.849)
  line L1664 (-0.0593, -74.674) -> (-0.0683, -74.7127)
  line L1665 (14.3512, -219.849) -> (14.3819, -219.8742)
  line L1666 (0.0978, -74.4019) -> (0.0706, -74.4308)
  line L1667 (19.8738, -174.5988) -> (19.8574, -174.5626)